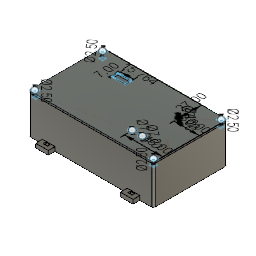
3d_enclosure_model_2409 v1 (Autodesk Fusion 360 design; units mm, degrees)
Autodesk Fusion 360 part; units mm, degrees
note: some values were not read from the file. Set by a fixed rule: which sketch regions a step uses.
sketch "Sketch1" plane through (0, 0, 0) normal (0, 0, 1) x (1, 0, 0)
  line L0 (144.999936, 0) -> (144.999936, 85) construction
  line L1 (144.999936, 85) -> (0, 85) construction
  line L2 (0, 85) -> (0, 0) construction
  line L3 (-1, -1) -> (145.999936, -1)
  line L4 (145.999936, -1) -> (145.999936, 86)
  line L5 (145.999936, 86) -> (-1, 86)
  line L6 (-1, 86) -> (-1, -1)
  circle A0 centre (71.000001, 46.000001) radius 3
  circle A1 centre (71.000001, 18) radius 3
  circle A2 centre (101.000002, 12) radius 3
  circle A3 centre (18, 12) radius 3
  line L7 (5, 80.000001) -> (0, 80.000001)
  line L8 (0, 80.000001) -> (0, 85)
  line L9 (0, 85) -> (5, 85)
  line L10 (5, 85) -> (5, 80.000001)
  line L11 (0, 5) -> (5, 5)
  line L12 (5, 5) -> (5, 0)
  line L13 (5, 0) -> (0, 0)
  line L14 (0, 0) -> (0, 5)
  line L15 (144.999936, 0) -> (140.000002, 0)
  line L16 (140.000002, 0) -> (140.000002, 5)
  line L17 (140.000002, 5) -> (144.999936, 5)
  line L18 (144.999936, 5) -> (144.999936, 0)
  circle A4 centre (142.499969, 2.5) radius 1.25
  circle A5 centre (2.5, 2.5) radius 1.25
  circle A6 centre (2.5, 82.500001) radius 1.25
  line L19 (140.01018, 85) -> (144.999936, 85)
  line L20 (144.999936, 85) -> (144.999936, 80.022328)
  line L21 (144.999936, 80.022328) -> (140.01018, 80.022328)
  line L22 (140.01018, 80.022328) -> (140.01018, 85)
  circle A7 centre (142.505058, 82.511164) radius 1.25
  line L23 (5, 80.000001) -> (1, 80.000001)
  line L24 (1, 80.000001) -> (1, 84.000001)
  line L25 (1, 84.000001) -> (5, 84.000001)
  line L26 (5, 84.000001) -> (5, 80.000001)
  line L27 (5, 5) -> (1, 5)
  line L28 (1, 5) -> (1, 1)
  line L29 (1, 1) -> (5, 1)
  line L30 (5, 1) -> (5, 5)
  line L31 (140.000002, 5) -> (144.000002, 5)
  line L32 (144.000002, 5) -> (144.000002, 1)
  line L33 (144.000002, 1) -> (140.000002, 1)
  line L34 (140.000002, 1) -> (140.000002, 5)
  line L35 (140.01018, 80.022328) -> (144.000002, 80.022328)
  line L36 (144.000002, 80.022328) -> (144.000002, 84.000001)
  line L37 (144.000002, 84.000001) -> (140.01018, 84.000001)
  line L38 (140.01018, 84.000001) -> (140.01018, 80.022328)
  dimension "d1" = 85
  dimension "d10" = 144.999936
  dimension "d112" = 6
  dimension "d113" = 6
  dimension "d114" = 6
  dimension "d115" = 6
  dimension "d231" = 2.5
  dimension "d232" = 2.5
  dimension "d233" = 2.5
  dimension "d234" = 2.5
  constraint vertical L0
  constraint horizontal L1
  constraint vertical L2
  constraint coincident L2.end L13.end
  constraint horizontal L7
  constraint vertical L8
  constraint horizontal L9
  constraint vertical L10
  constraint horizontal L11
  constraint vertical L12
  constraint horizontal L13
  constraint vertical L14
  constraint coincident L2 L11.start
  constraint horizontal L15
  constraint vertical L16
  constraint horizontal L17
  constraint vertical L18
  constraint horizontal L19
  constraint vertical L20
  constraint horizontal L21
  constraint vertical L22
  constraint horizontal L23
  constraint vertical L24
  constraint horizontal L25
  constraint vertical L26
  constraint horizontal L27
  constraint vertical L28
  constraint horizontal L29
  constraint vertical L30
  constraint horizontal L31
  constraint vertical L32
  constraint horizontal L33
  constraint vertical L34
  constraint horizontal L35
  constraint vertical L36
  constraint horizontal L37
  constraint vertical L38
  constraint parallel L0 L4
  constraint parallel L1 L5
  constraint parallel L2 L6
  measures "d1" distance of L2.end L1.end
  measures "d112" diameter of A0
  measures "d113" diameter of A1
  measures "d114" diameter of A2
  measures "d115" diameter of A3
  measures "d231" diameter of A4
  measures "d232" diameter of A5
  measures "d233" diameter of A6
  measures "d234" diameter of A7
extrude "Extrude22" add sketch "Sketch1" along normal blind 47 contours L3 L4 L5 L6 | A0 | A1 | A2 | A3 | L7 L10 L23 L24 L25 L26 | L7 L8 L9 L10 L24 L25 | L11 L12 L13 L14 L28 L29 | L11 L12 L27 L28 L29 L30 | L15 L16 L17 L18 L32 L33 | L16 L17 L31 L32 L33 L34 | A4 | A5 | A6 | L19 L20 L21 L22 L36 L37 | L21 L22 L35 L36 L37 L38 | A7 picked at (30.709844, 47.079917) picked at (71.820915, 46.965015) picked at (70.25578, 18.531131) picked at (100.25578, 12.531131) picked at (18.790611, 11.067645) picked at (4.57868, 82.104567) picked at (0.333333, 83.000001) picked at (2, 0.333333) picked at (4.57868, 2.895434) picked at (142.99998, 0.333333) picked at (140.421312, 2.895434) picked at (142.805408, 2.783405) picked at (2.407283, 2.869508) picked at (2.531138, 83.384936) picked at (143.003373, 84.666667) picked at (140.429793, 82.11573) picked at (142.160792, 82.152245) makes body 1
ref_plane "WorkPlane2" through (72.499968, 42.5, 45) normal (0, 0, 1) x (1, 0, 0)
fillet "Fillet2" radius 2 4 edges at (-1, -1, 23.5) (-1, 86, 23.5) (145.999936, -1, 23.5) (145.999936, 86, 23.5) on bodies 1
split "Split2" by plane through (72.499968, 42.5, 45) normal (0, 0, 1) bodies 1 makes body 2 at (48.666645, 28, 47)
shell "Shell2" thickness 2 removed faces 1 at (96.333291, 28, 45) on bodies 1
extrude "Extrude27" add sketch "Sketch1" along normal blind 6 contours A0 | A1 | A2 | A3 picked at (71.820915, 46.965015) picked at (70.25578, 18.531131) picked at (100.25578, 12.531131) picked at (18.790611, 11.067645) bodies 1
hole "Hole11" at (71.000001, 46.000001, 6) direction (0, 0, -1) diameter 2.5 depth 5 tip angle 180 bodies 1
hole "Hole12" at (71.000001, 18, 6) direction (0, 0, -1) diameter 2.5 depth 5 tip angle 180 bodies 1
hole "Hole13" at (101.000002, 12, 6) direction (0, 0, -1) diameter 2.5 depth 5 tip angle 180 bodies 1
hole "Hole15" at (18, 12, 6) direction (0, 0, -1) diameter 2.5 depth 5 tip angle 180 bodies 1
sketch "Sketch6" plane through (0, 0, 47) normal (0, 0, 1) x (-1, 0, 0)
  arc A0 (-145.999936, -84) -> (-143.999936, -86) centre (-143.999936, -84) ccw
  line L0 (-143.999936, -86) -> (-1, -86)
  arc A1 (-1, -86) -> (1, -84) centre (-1, -84) ccw
  line L1 (1, -84) -> (1, -1)
  arc A2 (1, -1) -> (-1, 1) centre (-1, -1) ccw
  line L2 (-1, 1) -> (-143.999936, 1)
  arc A3 (-143.999936, 1) -> (-145.999936, -1) centre (-143.999936, -1) ccw
  line L3 (-145.999936, -1) -> (-145.999936, -84)
  circle A4 centre (-113.000002, -19) radius 3.5
  circle A5 centre (-100.999936, -19) radius 3.5
  line L4 (-34.000001, -69.000001) -> (-49.764214, -69.000001)
  line L5 (-49.764214, -69.000001) -> (-49.764214, -62.000001)
  line L6 (-49.764214, -62.000001) -> (-34.000001, -62.000001)
  line L7 (-34.000001, -62.000001) -> (-34.000001, -69.000001)
  circle A6 centre (-115.999936, -59) radius 1.3
  line L8 (0, -85.000001) -> (-5, -85.000001)
  line L9 (-5, -85.000001) -> (-5, -80.000001)
  line L10 (-5, -80.000001) -> (0, -80.000001)
  line L11 (0, -80.000001) -> (0, -85.000001)
  circle A7 centre (-2.5, -82.500001) radius 1.25
  line L12 (0, -5) -> (-5, -5)
  line L13 (-5, -5) -> (-5, 0)
  line L14 (-5, 0) -> (0, 0)
  line L15 (0, 0) -> (0, -5)
  circle A8 centre (-2.5, -2.5) radius 1.25
  line L16 (-145.000002, 0) -> (-140.000002, 0)
  line L17 (-140.000002, 0) -> (-140.000002, -5)
  line L18 (-140.000002, -5) -> (-145.000002, -5)
  line L19 (-145.000002, -5) -> (-145.000002, 0)
  circle A9 centre (-142.500002, -2.5) radius 1.25
  line L20 (-140.000002, -85.000001) -> (-145.000002, -85.000001)
  line L21 (-145.000002, -85.000001) -> (-145.000002, -80.000001)
  line L22 (-145.000002, -80.000001) -> (-140.000002, -80.000001)
  line L23 (-140.000002, -80.000001) -> (-140.000002, -85.000001)
  circle A10 centre (-142.500002, -82.500001) radius 1.25
  circle A11 centre (-115.999936, -59) radius 2
  dimension "d192" = 7
  dimension "d194" = 7
  dimension "d210" = 7
  dimension "d215" = 15.764213
  dimension "d218" = 2.6
  dimension "d237" = 2.5
  dimension "d238" = 2.5
  dimension "d239" = 2.5
  dimension "d240" = 2.5
  dimension "d290" = 27
  dimension "d291" = 30
  dimension "d292" = 45
  dimension "d293" = 4
  constraint horizontal L4
  constraint vertical L5
  constraint horizontal L6
  constraint vertical L7
  constraint horizontal L8
  constraint vertical L9
  constraint horizontal L10
  constraint vertical L11
  constraint horizontal L12
  constraint vertical L13
  constraint horizontal L14
  constraint vertical L15
  constraint horizontal L16
  constraint vertical L17
  constraint horizontal L18
  constraint vertical L19
  constraint horizontal L20
  constraint vertical L21
  constraint horizontal L22
  constraint vertical L23
  constraint concentric A6 A11
  measures "d192" diameter of A4
  measures "d194" diameter of A5
  measures "d218" diameter of A6
  measures "d237" diameter of A7
  measures "d238" diameter of A8
  measures "d239" diameter of A9
  measures "d240" diameter of A10
  measures "d293" diameter of A11
extrude "Extrude48" cut sketch "Sketch6" against normal blind 3 contours A4 | A5 | L4 L5 L6 L7 | A6 picked at (-111.885167, -19.343881) picked at (-99.885101, -19.343881) picked at (-39.254738, -66.666668) picked at (-115.6419, -59.373275) bodies 2
extrude "Extrude49" add sketch "Sketch1" along normal blind 45 contours L7 L10 L23 L24 L25 L26 | L7 L8 L9 L10 L24 L25 | L11 L12 L13 L14 L28 L29 | L11 L12 L27 L28 L29 L30 | L15 L16 L17 L18 L32 L33 | L16 L17 L31 L32 L33 L34 | L19 L20 L21 L22 L36 L37 | L21 L22 L35 L36 L37 L38 picked at (4.57868, 82.104567) picked at (0.333333, 83.000001) picked at (2, 0.333333) picked at (4.57868, 2.895434) picked at (142.99998, 0.333333) picked at (140.421312, 2.895434) picked at (143.003373, 84.666667) picked at (140.429793, 82.11573) bodies 1
extrude "Extrude50" cut sketch "Sketch6" against normal blind 2 contours A7 | A8 | A9 | A10 picked at (-2.217461, -81.870639) picked at (-2.495612, -2.171219) picked at (-142.75979, -2.258953) picked at (-142.844268, -82.85892) bodies 2
extrude "Extrude51" add sketch "Sketch1" along normal blind 10 contours A6 picked at (2.531138, 83.384936) bodies 1
sketch "Sketch13" plane through (0, -1, 0) normal (0, -1, 0) x (1, 0, 0)
  line L0 (143.999936, 45) -> (1, 45)
  line L1 (1, 45) -> (1, 0)
  line L2 (1, 0) -> (143.999936, 0)
  line L3 (143.999936, 0) -> (143.999936, 45)
  line L4 (15, 0) -> (30, 0)
  line L5 (30, 0) -> (30, 5)
  line L6 (30, 5) -> (15, 5)
  line L7 (15, 5) -> (15, 0)
  line L8 (130, 5) -> (115.000002, 5)
  line L9 (115.000002, 5) -> (115.000002, 0)
  line L10 (115.000002, 0) -> (130, 0)
  line L11 (130, 0) -> (130, 5)
  dimension "d288" = 5
  dimension "d289" = 15
  constraint horizontal L4
  constraint vertical L5
  constraint horizontal L6
  constraint vertical L7
  constraint horizontal L8
  constraint vertical L9
  constraint horizontal L10
  constraint vertical L11
  constraint coincident L2 L4.start
  measures "d288" distance of L4.start L6.end
  measures "d289" distance of L5.end L6.end
extrude "Extrude63" add sketch "Sketch13" along normal blind 8 contours L2 L8 L9 L10 L11 | L2 L4 L5 L6 L7 picked at (125.000001, 1.666667) picked at (20, 3.333333) bodies 1
sketch "Sketch14" plane through (0, 86, 0) normal (0, 1, 0) x (-1, 0, 0)
  line L0 (-1, 45) -> (-143.999936, 45)
  line L1 (-143.999936, 45) -> (-143.999936, 0)
  line L2 (-143.999936, 0) -> (-1, 0)
  line L3 (-1, 0) -> (-1, 45)
  line L4 (-130, 0) -> (-115, 0)
  line L5 (-115, 0) -> (-115, 5)
  line L6 (-115, 5) -> (-130, 5)
  line L7 (-130, 5) -> (-130, 0)
  line L8 (-15, 5) -> (-30, 5)
  line L9 (-30, 5) -> (-30, 0)
  line L10 (-30, 0) -> (-15, 0)
  line L11 (-15, 0) -> (-15, 5)
  constraint horizontal L4
  constraint vertical L5
  constraint horizontal L6
  constraint vertical L7
  constraint horizontal L8
  constraint vertical L9
  constraint horizontal L10
  constraint vertical L11
  constraint coincident L2 L4.start
  constraint coincident L2 L9.end
extrude "Extrude54" add sketch "Sketch13" along normal blind 8 contours L2 L8 L9 L10 L11 | L2 L4 L5 L6 L7 picked at (125.000001, 1.666667) picked at (20, 3.333333) bodies 1
extrude "Extrude55" add sketch "Sketch14" along normal blind 8 contours L2 L8 L9 L10 L11 | L2 L4 L5 L6 L7 picked at (-20, 1.666667) picked at (-125, 3.333333) bodies 1
ref_plane "WorkPlane5" through (72.499968, 42.5, 40) normal (0, 0, 1) x (1, 0, 0)
extrude "Extrude62" cut sketch "Sketch1" along normal blind 36 from surface at 2 contours L7 L10 L23 L24 L25 L26 | L11 L12 L27 L28 L29 L30 | L16 L17 L31 L32 L33 L34 | A4 | A5 | A6 | L21 L22 L35 L36 L37 L38 | A7 picked at (4.57868, 82.104567) picked at (4.57868, 2.895434) picked at (140.421312, 2.895434) picked at (142.805408, 2.783405) picked at (2.407283, 2.869508) picked at (2.531138, 83.384936) picked at (140.429793, 82.11573) picked at (142.160792, 82.152245) bodies 1
sketch "Sketch21" plane through (0, 80.000001, 0) normal (0, -1, 0) x (1, 0, 0)
  line L0 (1, 38) -> (5, 38)
  line L1 (5, 38) -> (5, 45)
  line L2 (5, 45) -> (1, 45)
  line L3 (1, 45) -> (1, 38)
  line L4 (1, 38) -> (1, 33)
  line L5 (5, 38) -> (1, 33)
  dimension "d275" = 5
  constraint coincident L0.start L3.end
  constraint perpendicular L0 L4
  constraint coincident L0.end L1.start
  measures "d275" distance of L0.start L4.end
extrude "Extrude64" add sketch "Sketch21" against normal blind 4 contours L0 L4 L5 picked at (2.333333, 36.333333) bodies 1
sketch "Sketch23" plane through (0, 80.022328, 0) normal (0, -1, 0) x (1, 0, 0)
  line L0 (140.01018, 38) -> (143.999936, 38)
  line L1 (143.999936, 38) -> (143.999936, 45)
  line L2 (143.999936, 45) -> (140.01018, 45)
  line L3 (140.01018, 45) -> (140.01018, 38)
  line L4 (144.000002, 2) -> (144.000002, 38)
  line L5 (143.999936, 45) -> (144.000002, 33)
  line L6 (144.000002, 33) -> (140.01018, 38)
extrude "Extrude65" add sketch "Sketch23" against normal blind 4 contours L0 L4 L5 L6 picked at (142.67004, 36.333333) bodies 1
sketch "Sketch24" plane through (0, 5, 0) normal (0, 1, 0) x (-1, 0, 0)
  line L0 (-143.999936, 38) -> (-140.000002, 38)
  line L1 (-140.000002, 38) -> (-140.000002, 45)
  line L2 (-140.000002, 45) -> (-143.999936, 45)
  line L3 (-143.999936, 45) -> (-143.999936, 38)
  line L4 (-144.000002, 2) -> (-144.000002, 38)
  line L5 (-143.999936, 45) -> (-144.000002, 33)
  line L6 (-144.000002, 33) -> (-140.000002, 38)
extrude "Extrude66" add sketch "Sketch24" against normal blind 4 contours L0 L4 L5 L6 picked at (-142.666628, 36.333333) bodies 1
sketch "Sketch28" plane through (0, 5, 0) normal (0, 1, 0) x (-1, 0, 0)
  line L0 (-5, 38) -> (-1, 38)
  line L1 (-1, 38) -> (-1, 45)
  line L2 (-1, 45) -> (-5, 45)
  line L3 (-5, 45) -> (-5, 38)
  line L4 (-1, 38) -> (-1, 33)
  line L5 (-1, 33) -> (-5, 38)
  dimension "d283" = 5
  constraint coincident L0.end L1.start
  constraint perpendicular L0 L4
  constraint coincident L0.start L3.end
  measures "d283" distance of L0.end L4.end
extrude "Extrude67" add sketch "Sketch28" against normal blind 4 contours L0 L4 L5 picked at (-2.333333, 36.333333) bodies 1
sketch "Sketch29" plane through (0, 0, 5) normal (0, 0, 1) x (-1, 0, 0)
  line L0 (-30, 1) -> (-15, 1)
  line L1 (-15, 1) -> (-15, 9)
  line L2 (-15, 9) -> (-30, 9)
  line L3 (-30, 9) -> (-30, 1)
  line L4 (-20, 2) -> (-25, 2)
  line L5 (-25, 2) -> (-25, 5)
  line L6 (-25, 5) -> (-20, 5)
  line L7 (-20, 5) -> (-20, 2)
  line L8 (-120.000002, 2) -> (-125.000002, 2)
  line L9 (-125.000002, 2) -> (-125.000002, 5)
  line L10 (-125.000002, 5) -> (-120.000002, 5)
  line L11 (-120.000002, 5) -> (-120.000002, 2)
  constraint horizontal L4
  constraint vertical L5
  constraint horizontal L6
  constraint vertical L7
  constraint horizontal L8
  constraint vertical L9
  constraint horizontal L10
  constraint vertical L11
sketch "Sketch30" plane through (0, 0, 5) normal (0, 0, 1) x (-1, 0, 0)
  line L0 (-15, -86) -> (-30, -86)
  line L1 (-30, -86) -> (-30, -94)
  line L2 (-30, -94) -> (-15, -94)
  line L3 (-15, -94) -> (-15, -86)
  line L4 (-25, -87.000001) -> (-20, -87.000001)
  line L5 (-20, -87.000001) -> (-20, -90.000001)
  line L6 (-20, -90.000001) -> (-25, -90.000001)
  line L7 (-25, -90.000001) -> (-25, -87.000001)
  line L8 (-125.000002, -87.000001) -> (-120.000002, -87.000001)
  line L9 (-120.000002, -87.000001) -> (-120.000002, -90.000001)
  line L10 (-120.000002, -90.000001) -> (-125.000002, -90.000001)
  line L11 (-125.000002, -90.000001) -> (-125.000002, -87.000001)
  constraint horizontal L4
  constraint vertical L5
  constraint horizontal L6
  constraint vertical L7
  constraint horizontal L8
  constraint vertical L9
  constraint horizontal L10
  constraint vertical L11
extrude "Extrude68" cut sketch "Sketch29" sketch "Sketch30" against normal blind 5 contours L4 L5 L6 L7 | L8 L9 L10 L11 picked at (-21.666667, 3) picked at (-121.666668, 3) of sketch 2 contours L4 L5 L6 L7 | L8 L9 L10 L11 picked at (-23.333334, -88.000001) picked at (-123.333335, -88.000001) bodies 1
extrude "Extrude69" cut sketch "Sketch6" against normal blind 3 contours A11 picked at (-117.221953, -57.730589) bodies 2
sketch "Sketch17" plane through (0, 0, 0) normal (0, 0, -1) x (-1, 0, 0)
  line L0 (-1, 86) -> (-15, 86)
  line L1 (-130, 94) -> (-130, 86)
  line L2 (-15, 94) -> (-30, 94)
  line L3 (-115, 86) -> (-115, 94)
  line L4 (-125.000002, -87.000001) -> (-120.000002, -87.000001)
  line L5 (-120.000002, -87.000001) -> (-120.000002, -90.000001)
  line L6 (-120.000002, -90.000001) -> (-125.000002, -90.000001)
  line L7 (-125.000002, -90.000001) -> (-125.000002, -87.000001)
  line L8 (-20, 90.000001) -> (-20, 87.000001)
  line L9 (-20, 87.000001) -> (-25, 87.000001)
  line L10 (-25, 87.000001) -> (-25, 90.000001)
  line L11 (-25, 90.000001) -> (-20, 90.000001)
  line L12 (-25, -5) -> (-25, -2)
  line L13 (-25, -2) -> (-20, -2)
  line L14 (-20, -2) -> (-20, -5)
  line L15 (-20, -5) -> (-25, -5)
  line L16 (-125.000002, -5) -> (-125.000002, -2)
  line L17 (-125.000002, -2) -> (-120.000002, -2)
  line L18 (-120.000002, -2) -> (-120.000002, -5)
  line L19 (-120.000002, -5) -> (-125.000002, -5)
  line L20 (-120.000002, 90.000001) -> (-120.000002, 87.000001)
  line L21 (-120.000002, 87.000001) -> (-125.000002, 87.000001)
  line L22 (-125.000002, 87.000001) -> (-125.000002, 90.000001)
  line L23 (-125.000002, 90.000001) -> (-120.000002, 90.000001)
  line L24 (-115.000002, -1) -> (-30, -1)
  line L25 (-30, -1) -> (-30, -9)
  line L26 (-30, -9) -> (-15, -9)
  line L27 (-15, -9) -> (-15, -1)
  line L28 (-15, -1) -> (-1, -1)
  arc A0 (-1, -1) -> (1, 1) centre (-1, 1) ccw
  line L29 (1, 1) -> (1, 84)
  arc A1 (1, 84) -> (-1, 86) centre (-1, 84) ccw
  line L30 (-15, 86) -> (-15, 94)
  line L31 (-30, 94) -> (-30, 86)
  line L32 (-30, 86) -> (-115, 86)
  line L33 (-115, 94) -> (-130, 94)
  line L34 (-130, 86) -> (-143.999936, 86)
  arc A2 (-143.999936, 86) -> (-145.999936, 84) centre (-143.999936, 84) ccw
  line L35 (-145.999936, 84) -> (-145.999936, 1)
  arc A3 (-145.999936, 1) -> (-143.999936, -1) centre (-143.999936, 1) ccw
  line L36 (-143.999936, -1) -> (-130, -1)
  line L37 (-130, -1) -> (-130, -9)
  line L38 (-130, -9) -> (-115.000002, -9)
  line L39 (-115.000002, -9) -> (-115.000002, -1)
  constraint horizontal L4
  constraint vertical L5
  constraint horizontal L6
  constraint vertical L7
sketch "Sketch18" plane through (0, 0, 0) normal (0, 0, -1) x (-1, 0, 0)
  line L0 (-1, 86) -> (-15, 86)
  line L1 (-30, 94) -> (-30, 86)
  line L2 (-15, 94) -> (-30, 94)
  line L3 (-15, 86) -> (-15, 94)
  line L4 (-25, -87.000001) -> (-20, -87.000001)
  line L5 (-20, -87.000001) -> (-20, -90.000001)
  line L6 (-20, -90.000001) -> (-25, -90.000001)
  line L7 (-25, -90.000001) -> (-25, -87.000001)
  line L8 (-20, 90.000001) -> (-20, 87.000001)
  line L9 (-20, 87.000001) -> (-25, 87.000001)
  line L10 (-25, 87.000001) -> (-25, 90.000001)
  line L11 (-25, 90.000001) -> (-20, 90.000001)
  line L12 (-25, -5) -> (-25, -2)
  line L13 (-25, -2) -> (-20, -2)
  line L14 (-20, -2) -> (-20, -5)
  line L15 (-20, -5) -> (-25, -5)
  line L16 (-125.000002, -5) -> (-125.000002, -2)
  line L17 (-125.000002, -2) -> (-120.000002, -2)
  line L18 (-120.000002, -2) -> (-120.000002, -5)
  line L19 (-120.000002, -5) -> (-125.000002, -5)
  line L20 (-120.000002, 90.000001) -> (-120.000002, 87.000001)
  line L21 (-120.000002, 87.000001) -> (-125.000002, 87.000001)
  line L22 (-125.000002, 87.000001) -> (-125.000002, 90.000001)
  line L23 (-125.000002, 90.000001) -> (-120.000002, 90.000001)
  line L24 (-115.000002, -1) -> (-30, -1)
  line L25 (-30, -1) -> (-30, -9)
  line L26 (-30, -9) -> (-15, -9)
  line L27 (-15, -9) -> (-15, -1)
  line L28 (-15, -1) -> (-1, -1)
  arc A0 (-1, -1) -> (1, 1) centre (-1, 1) ccw
  line L29 (1, 1) -> (1, 84)
  arc A1 (1, 84) -> (-1, 86) centre (-1, 84) ccw
  line L30 (-30, 86) -> (-115, 86)
  line L31 (-115, 86) -> (-115, 94)
  line L32 (-115, 94) -> (-130, 94)
  line L33 (-130, 94) -> (-130, 86)
  line L34 (-130, 86) -> (-143.999936, 86)
  arc A2 (-143.999936, 86) -> (-145.999936, 84) centre (-143.999936, 84) ccw
  line L35 (-145.999936, 84) -> (-145.999936, 1)
  arc A3 (-145.999936, 1) -> (-143.999936, -1) centre (-143.999936, 1) ccw
  line L36 (-143.999936, -1) -> (-130, -1)
  line L37 (-130, -1) -> (-130, -9)
  line L38 (-130, -9) -> (-115.000002, -9)
  line L39 (-115.000002, -9) -> (-115.000002, -1)
  constraint horizontal L4
  constraint vertical L5
  constraint horizontal L6
  constraint vertical L7
extrude "Extrude58" cut sketch "Sketch17" against normal blind 5 contours L4 L5 L6 L7 picked at (-123.333335, -88.000001) bodies 1
extrude "Extrude59" cut sketch "Sketch18" against normal blind 5 contours L4 L5 L6 L7 picked at (-23.333334, -88.000001) bodies 1
ref_plane "WorkPlane4" through (72.499968, 42.5, 40) normal (0, 0, 1) x (1, 0, 0)
sketch "Sketch19" plane through (72.499968, 42.5, 40) normal (0, 0, 1) x (1, 0, 0)
  line L0 (67.500001, -37.500001) -> (71.500001, -37.500001)
  line L1 (71.500001, -37.500001) -> (71.500001, -41.500001)
  line L2 (71.500001, -41.500001) -> (67.500001, -41.500001)
  line L3 (67.500001, -41.500001) -> (67.500001, -37.500001)
  line L4 (67.500001, 37.500001) -> (71.500001, 37.500001)
  line L5 (71.500001, 37.500001) -> (71.500001, 41.500001)
  line L6 (71.500001, 41.500001) -> (67.500001, 41.500001)
  line L7 (67.500001, 41.500001) -> (67.500001, 37.500001)
  line L8 (-67.500001, 37.500001) -> (-71.500001, 37.500001)
  line L9 (-71.500001, 37.500001) -> (-71.500001, 41.500001)
  line L10 (-71.500001, 41.500001) -> (-67.500001, 41.500001)
  line L11 (-67.500001, 41.500001) -> (-67.500001, 37.500001)
  line L12 (-67.500001, -37.500001) -> (-71.499613, -37.500001)
  line L13 (-71.499613, -37.500001) -> (-71.499613, -41.500001)
  line L14 (-71.499613, -41.500001) -> (-67.500001, -41.500001)
  line L15 (-67.500001, -41.500001) -> (-67.500001, -37.500001)
  dimension "d266" = 4
  constraint horizontal L0
  constraint vertical L1
  constraint horizontal L2
  constraint vertical L3
  constraint horizontal L4
  constraint vertical L5
  constraint horizontal L6
  constraint vertical L7
  constraint horizontal L8
  constraint vertical L9
  constraint horizontal L10
  constraint vertical L11
  constraint horizontal L12
  constraint vertical L13
  constraint horizontal L14
  constraint vertical L15
extrude "Extrude61" cut sketch "Sketch19" against normal blind 38 contours L0 L1 L2 L3 | L4 L5 L6 L7 | L8 L9 L10 L11 | L12 L13 L14 L15 picked at (68.833334, -38.833334) picked at (68.833334, 40.166667) picked at (-68.833334, 38.833334) picked at (-70.166409, -38.833334) bodies 1
extrude "Extrude60" cut sketch "Sketch19" against normal blind 38 contours L0 L1 L2 L3 | L4 L5 L6 L7 picked at (68.833334, -38.833334) picked at (68.833334, 40.166667) bodies 1
sketch "Sketch9" plane through (0, -1, 0) normal (0, -1, 0) x (1, 0, 0)
  line L0 (143.999936, 45) -> (1, 45)
  line L1 (1, 45) -> (1, 0)
  line L2 (130, 0) -> (143.999936, 0)
  line L3 (143.999936, 0) -> (143.999936, 45)
  line L4 (115, 15) -> (130, 15)
  line L5 (130, 15) -> (130, 10)
  line L6 (130, 10) -> (115, 10)
  line L7 (115, 10) -> (115, 15)
  line L8 (15, 15) -> (30, 15)
  line L9 (30, 15) -> (30, 10)
  line L10 (30, 10) -> (15, 10)
  line L11 (15, 10) -> (15, 15)
  line L12 (115.000002, 0) -> (115.000002, 5)
  line L13 (115.000002, 5) -> (130, 5)
  line L14 (130, 5) -> (130, 0)
  line L15 (1, 0) -> (15, 0)
  line L16 (15, 0) -> (15, 5)
  line L17 (15, 5) -> (30, 5)
  line L18 (30, 5) -> (30, 0)
  line L19 (30, 0) -> (115.000002, 0)
  constraint horizontal L4
  constraint vertical L5
  constraint horizontal L6
  constraint vertical L7
  constraint horizontal L8
  constraint vertical L9
  constraint horizontal L10
  constraint vertical L11
named bodies: "Bottom", "Top"
